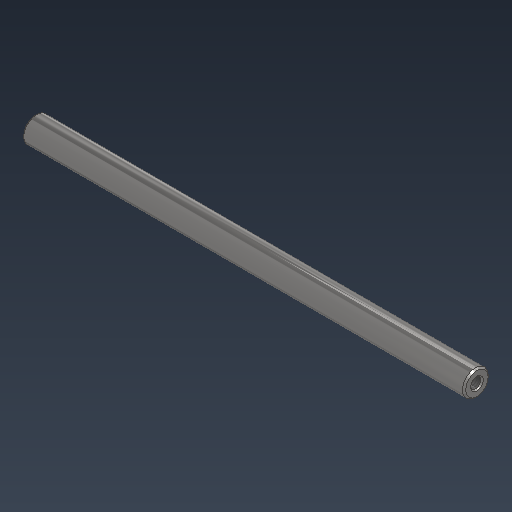
# Autodesk Inventor part: SFHRW8-137-M4-N4_s
Saved by Autodesk Inventor 2021 (Build 250183000, 183)
## iProperties
Category: PARTsolutions
Company: MISUMI
Part Number: SFHRW8-137-M4-N4_s
Material: 鋼、炭素鋼
Catalog Web Link: www.cadenas.de
Description: NSFMRW, SFMRW, PSFMRW, SSFMRW, NSFHRW, SFHRW, PSFHRW, PPSFHRW, SSFHRW, SSSFHRW, NSFRW, SFRW, PSFRW, PPSFRW, SSFRW, SSSFRW, HFRW, PHFRW_shaft-Rotary Shafts - Both Ends Tapped - Standard
Vendor: MISUMI
Document SubType Name: Modeling
Designer: partserver
Manufacturer: MISUMI
Mass: 52.2648 g
Surface Area: 37.9287 cm^2
Volume: 6.65793 cm^3
Density: 7.85 g/cm^3
Appearance: 半つや出し
PSOL_IDENT_0: {$CADENAS_DATA\23d-libs\misumi\metric\11_rotary_shafts\11_components\phfrw\phfrw.prj},556 {VTYP=3D},
PSOL_IDENT_1: {NB=SFHRW8-137-M4-N4_s},{LINA=SFHRW8-137-M4-N4},{NN=NSFMRW, SFMRW, PSFMRW, SSFMRW, NSFHRW, SFHRW, PS
PSOL_IDENT_2: FHRW, PPSFHRW, SSFHRW, SSSFHRW, NSFRW, SFRW, PSFRW, PPSFRW, SSFRW, SSSFRW, HFRW, PHFRW_shaft},{DATE=
PSOL_IDENT_3: 27.07.2021 05:05:18},{GEOMDATE=15.07.2021 04:13:12},{VERSION=},{LINEID=20},{WBVAR=TS,MAT,ST,ALT1,L,M
PSOL_IDENT_4: ,N,ALT2,KC,A,WKC,C,K,E,KZ,Z,ALT3,FC,GALT3,WFC,J,WALT3,V,ALT4,SFC,SGALT4,AG,ALT5,UC,ALT6,TA,TB,ALT31,
PSOL_IDENT_5: ALT34,TCJ,WTCJ,XT,ALT35,HCJ,WHCJ,XH},{WBNUMERIC=L,M,N,KC,A,WKC,C,K,E,KZ,Z,FC,GALT3,WFC,J,WALT3,V,SFC
PSOL_IDENT_6: ,SGALT4,AG,UC,TA,TB,TCJ,WTCJ,XT,HCJ,WHCJ,XH}  {NB=SFHRW8-137-M4-N4_s},{LINA=SFHRW8-137-M4-N4},{KT=DU
PSOL_IDENT_7: MMY},{PN=SFHRW8-137-M4-N4},{TYPE=SFHRW},{TS=H},{TSALG= 'M','h9 (Cold-drawn)','H','h7 (Ground)','','g
PSOL_IDENT_8: 6 (Ground)' },{MAT=S45C},{MATALG= 'S45C','S45C Equivalent', 'SUS304','304 Stainless Steel','SUS303','
PSOL_IDENT_9: 303 Stainless Steel' },{ST=BO},{STALG= '','-','BO','Black Oxide', 'ENP','Electroless Nickel Plating'
PSOL_IDENT_10: , 'HCP','Hard chrome plating' },{D=8},{ALT1=},{L=137.0},{LALG=[15:500/0.1]},{LMINALG=15},{LMIN=15},{
PSOL_IDENT_11: LMAX=500},{M=4},{MALG=2.6,3,4,5,6},{MMIN=2.6},{N=4},{NALG=2.6,3,4,5,6},{NMIN=2.6},{NMAX=6},{NMAXD=6}
PSOL_IDENT_12: ,{NALGMEQN=30},{NALGMGTN=30},{NALGMLTN=30},{PITCH=0.7},{PITCHM=0.7},{ALT2=},{ALT2ALG= '', 'w/o Key G
PSOL_IDENT_13: rooves','KC','with KC (Key Groove)','WKC','with WKC (Two Key Grooves)','KCWKC','with KC + WKC (Three
PSOL_IDENT_14: Key Grooves)','KZ','with KC + WKC + KZ (Four Key Grooves)' },{ALT2PN=},{KC=0.0},{KCALG=[0]},{KCMIN=
PSOL_IDENT_15: 0},{KCMAX=0},{A=0.0},{AALG=[0]},{AMIN=3},{AMAX=0},{WKC=0.0},{WKCALG=[0]},{WKCMIN=0},{WKCMAX=0},{C=0.
PSOL_IDENT_16: 0},{CALG=[0]},{CMIN=3},{CMAX=0},{K=0.0},{KALG=[0]},{KMIN=0},{KMAX=132},{E=0.0},{EALG=[0]},{EMIN=3},{
PSOL_IDENT_17: EMAX=100},{KZ=0.0},{KZALG=[0]},{KZMIN=139},{KZMAX=134},{Z=0.0},{ZALG=[0]},{ZMIN=3},{ZMAX=100},{BB=0}
PSOL_IDENT_18: ,{BBALT2=3},{TT=0.0},{TTALT2=1.8},{CIFKC=1.000},{CIFWKC=1.000},{CIFK=1.000},{CIFKZ=2.000},{PCUT3D=0.
PSOL_IDENT_19: 000},{QCUT3D=0.000},{ALT3=},{ALT3ALG= '', 'w/o Set Screw Flat','FC','with FC (Adds a Set Screw Flat)'
PSOL_IDENT_20: ,'WFC','with WFC (Adds Two Set Screw Flats)','FCWFC','with FC + WFC (Adds Three Set Screw Flats)' },
PSOL_IDENT_21: {ALT3PN=},{FC=0},{FCALG=[0]},{FCMIN=0},{FCMAX=136},{GALT3=0},{GALT3ALG=[0]},{GALT3MIN=1},{GALT3MAX=7
PSOL_IDENT_22: 0},{GALT3MAX2=70},{GALT3MAX3=70},{WFC=0},{WFCALG=[0]},{WFCMIN=0},{WFCMIN2=2},{WFCMAX=133},{WFCMAX2=-
PSOL_IDENT_23: 3},{WFCMAX3=-4},{J=0},{JALG=[0]},{JMIN=1},{JMAX=70},{JMAX2=-2},{JMAX3=-5},{WALT3=0},{WALT3ALG=[0]},{
PSOL_IDENT_24: WALT3MIN=0},{WALT3MIN2=139},{WALT3MAX=134},{WALT3MAX2=134},{V=0},{VALG=[0]},{VMIN=1},{VMAX=70},{VMAX
PSOL_IDENT_25: 2=70},{CIFFC=0},{ALT4=},{ALT4ALG= '', 'w/o SFC (2 Set Screw Flats (Angle Specified))', 'SFC'  , 'wit
PSOL_IDENT_26: h SFC (2 Set Screw Flats (Angle Specified))'},{ALT4PN=},{SFC=0},{SFCALG=[0]},{SFCMIN=0},{SFCMAX=136}
PSOL_IDENT_27: ,{SGALT4=0},{SGALT4ALG=[0]},{SGALT4MIN=1},{SGALT4MAX=70},{AG=0},{AGALG=[0]},{H=0.0},{CIFSFC=0},{ALT5=
PSOL_IDENT_28: },{ALT5ALG= '', 'w/o UC (Slit Cam Groove)', 'UC', 'with UC (Slit Cam Groove)'},{ALT5PN=},{UC=0},{UCA
PSOL_IDENT_29: LG=[0]},{UCMIN=1},{UCMAX=132},{DDALT5=0},{LL1=0},{ALT6=},{ALT6ALG= '','w/o Retaining Ring Groove','T
PSOL_IDENT_30: A','with TA (Retaining Ring Groove)','TB','with TB (Retaining Ring Groove)','TATB','with TA + TB (Tw
PSOL_IDENT_31: o Retaining Ring Grooves)' },{ALT6PN=},{TA=0.0},{TAALG=[0]},{TAMIN=2},{TAMAX=0},{TB=0.0},{TBALG=[0]}
PSOL_IDENT_32: ,{TBMIN=2},{TBMAX=0},{DDALT6=0.0},{MM=0.00},{ALT31=},{ALT31ALG= '', 'w/o Tapped Depth','MD','with MD
PSOL_IDENT_33: (Tapped Depth)','ND','with ND (Tapped Depth)','MDND','with MD + ND (Tapped Depth)' },{CIFALT31M=0},
PSOL_IDENT_34: {CIFALT31N=0},{ML=14},{NL=14},{ML3D1=8},{ML3D2=14},{NL3D1=8},{NL3D2=14},{CIFMN3D=0},{ALT34=},{ALT34A
PSOL_IDENT_35: LG= '', 'w/o Through Tapped','TCJ','with TCJ (Through Tapped One Location)','WTCJ','with WTCJ (Throu
PSOL_IDENT_36: gh Tapped Two Locations)' },{ALT34PN=},{TCJ=0},{TCJALG=0},{TCJMIN=18},{TCJMAX=66},{WTCJ=0},{WTCJALG=
PSOL_IDENT_37: 0},{WTCJMAX=111},{XT=0},{XTALG=0},{XTMIN=18},{XTMAX=129},{TM=-},{TM3D=4},{ALT35=},{ALT35ALG= '', 'w/
PSOL_IDENT_38: o Through Hole','HCJ','with HCJ (Through Hole One Location)','WHCJ','with WHCJ (Through Hole Two Loc
PSOL_IDENT_39: ations)' },{ALT35PN=},{HCJ=0},{HCJALG=0},{HCJMIN=18},{HCJMAX=66},{WHCJ=0},{WHCJALG=0},{WHCJMAX=111},
PSOL_IDENT_40: {XH=0},{XHALG=0},{XHMIN=18},{XHMAX=129},{HP=0},{HP3D=4},{ERRORPN=},{ERRORMALT2=OK},{ERRORMALT3=OK},{
PSOL_IDENT_41: ERRORMALT4=OK},{ERRORMALT5=OK},{ERRORMALT6=OK},{ERRORNALT2=OK},{ERRORNALT3=OK},{ERRORNALT4=OK},{ERRO
PSOL_IDENT_42: RNALT5=OK},{ERRORNALT6=OK},{ERRORALT23=OK},{ERRORALT24=OK},{ERRORALT25=OK},{ERRORALT26=OK},{ERRORALT
PSOL_IDENT_43: 34=OK},{ERRORALT35=OK},{ERRORALT36=OK},{ERRORALT45=OK},{ERRORALT46=OK},{ERRORALT56=OK},{ERRORALT234=
PSOL_IDENT_44: OK},{ERRORALT235=OK},{ERRORALT334=OK},{ERRORALT335=OK},{ERRORALT434=OK},{ERRORALT435=OK},{ERRORALT53
PSOL_IDENT_45: 4=OK},{ERRORALT535=OK},{ERRORALT634=OK},{ERRORALT635=OK}
NB: SFHRW8-137-M4-N4_s
NN: NSFMRW, SFMRW, PSFMRW, SSFMRW, NSFHRW, SFHRW, PSFHRW, PPSFHRW, SSFHRW, SSSFHRW, NSFRW, SFRW, PSFRW, PPSFRW, SSFRW, SSSFRW, HFRW, PHFRW_shaft
NT: Rotary Shafts - Both Ends Tapped - Standard
NBSYN: $PN._s
LINA: SFHRW8-137-M4-N4
CATALOG: Misumi
PN: SFHRW8-137-M4-N4
TS: h7 (Ground)
MAT: S45C Equivalent
ST: Black Oxide
D: 8
ALT1: w/o LKC (Changes L Tolerance)
L: 137
M: 4
N: 4
ALT2: w/o Key Grooves
KC: 0
A: 0
WKC: 0
C: 0
K: 0
E: 0
KZ: 0
Z: 0
BB: 0
TT: 0
ALT3: w/o Set Screw Flat
FC: 0
GALT3: 0
WFC: 0
J: 0
WALT3: 0
V: 0
ALT4: w/o SFC (2 Set Screw Flats (Angle Specified))
SFC: 0
SGALT4: 0
AG: 0
H: 0
ALT5: w/o UC (Slit Cam Groove)
UC: 0
DDALT5: 0
LL1: 0
ALT6: w/o Retaining Ring Groove
TA: 0
TB: 0
DDALT6: 0
MM: 0
ALT31: w/o Tapped Depth
ALT34: w/o Through Tapped
TCJ: 0
WTCJ: 0
XT: 0
TM: -
ALT35: w/o Through Hole
HCJ: 0
WHCJ: 0
XH: 0
HP: 0
SUPPLIER: MISUMI
ARTICLENO: SFHRW8-137-M4-N4_s
BOMINFO: SFHRW8-137-M4-N4
CREATOR: CADENAS GmbH
在庫数: 0.0
購入先: ミスミ
Title: SFHRW8-137-M4-N4
Author: Cadenas PARTsolutions
Comments: Rotary Shafts - Both Ends Tapped - Standard
Autodesk Inventor part; units mm, degrees
ref_plane "YZ Plane" through (0, 0, 0) normal (1, 0, 0) x (0, 1, 0)
ref_plane "XZ Plane" through (0, 0, 0) normal (0, 1, 0) x (-1, 0, 0)
ref_plane "XY Plane" through (0, 0, 0) normal (0, 0, 1) x (1, 0, 0)
sketch "Sketch_1" plane through (0, 0, 0) normal (0, 0, 1) x (1, 0, 0)
  line L0 (137, 0) -> (0, 0)
  line L1 (0, 0) -> (0, 3.5)
  line L2 (0, 3.5) -> (0.5, 4)
  line L3 (0.5, 4) -> (136.5, 4)
  line L4 (136.5, 4) -> (137, 3.5)
  line L5 (137, 3.5) -> (137, 0)
  line L6 (137, 0) -> (0, 0)
  constraints: 14 end point
revolve "Revolution1" add sketch "Sketch_1" angle 360 about axis through (137, 0, 0) along (1, 0, 0)
sketch "Sketch2" plane through (0, 0, 0) normal (-1, 0, 0) x (0, 0, 1)
  point P0 (0, 0)
hole "Hole1" at (0, 0, 0) direction (1, 0, 0) diameter 3.242 depth 13.0641 tip angle 120 countersink diameter 4 countersink angle 90 thread size "M4x0.7" class "6H" standard "ISO Metric profile"
sketch "Sketch3" plane through (137, 0, 0) normal (1, 0, 0) x (0, 0, -1)
  point P0 (0, 0)
hole "Hole2" at (137, 0, 0) direction (-1, 0, 0) diameter 3.242 depth 13.0641 tip angle 120 countersink diameter 4 countersink angle 90 thread size "M4x0.7" class "6H" standard "ISO Metric profile"
body "Solid1"
